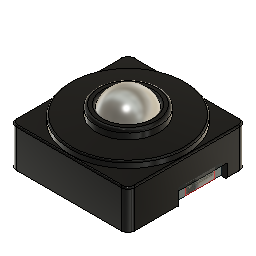
Pixart PAW3204 0A v2 (Autodesk Fusion 360 design; units mm, degrees)
Autodesk Fusion 360 part; units mm, degrees
note: some values were not read from the file. Set by a fixed rule: which sketch regions a step uses.
sketch "Skizze1" plane through (0, 0, 0) normal (0, 0, 1) x (1, 0, 0)
  line L0 (8.5, -8.5) -> (-8.5, -8.5)
  line L1 (-8.5, -8.5) -> (-8.5, 8.5)
  line L2 (-8.5, 8.5) -> (8.5, 8.5)
  line L3 (8.5, 8.5) -> (8.5, -8.5)
  line L4 (8.5, -8.5) -> (-8.5, 8.5) construction
  line L5 (-8.5, -8.5) -> (8.5, 8.5) construction
  dimension "d1" = 17
  dimension "d2" = 17
  constraint horizontal L0
  constraint perpendicular L0 L1
  constraint parallel L0 L2
  constraint parallel L1 L3
  constraint coincident L4 origin
  constraint coincident L5 origin
  measures "d1" distance of L1.end L2.end
  measures "d2" distance of L0.end L1.end
extrude "Extrusion1" add sketch "Skizze1" along normal blind 5.75 makes body 1
sketch "Skizze2" plane through (0, 0, 5.75) normal (0, 0, 1) x (-1, 0, 0)
  line L0 (-8.5, -8.5) -> (8.5, -8.5)
  line L1 (8.5, -8.5) -> (8.5, 8.5)
  line L2 (8.5, 8.5) -> (-8.5, 8.5)
  line L3 (-8.5, 8.5) -> (-8.5, -8.5)
  circle A0 centre (0, 0) radius 8.25
  dimension "d5" = 16.5
  constraint coincident A0.centre origin
  measures "d5" diameter of A0
extrude "Extrusion2" add sketch "Skizze2" along normal blind 0.9 contours A0 bodies 1
sketch "Skizze3" plane through (0, 0, 6.65) normal (0, 0, 1) x (-1, 0, 0)
  circle A0 centre (0, 0) radius 8.25
  circle A1 centre (0, 0) radius 4.5
  dimension "d8" = 9
  constraint coincident A0.centre A1.centre
  measures "d8" diameter of A1
extrude "Extrusion3" add sketch "Skizze3" along normal blind 1.25 contours A1 bodies 1
sketch "Skizze4" plane through (0, 0, 0) normal (0, 1, 0) x (1, 0, 0)
  circle A0 centre (0, -6.4) radius 3.5
  line L0 (-8.5, 0) -> (8.5, 0)
  line L1 (0, 0) -> (0, -9.9) construction
  line L2 (0, -9.9) -> (0, -2.9)
  dimension "d11" = 7
  dimension "d12" = 9.9
  constraint coincident L1.start origin
  constraint coincident A0 L1.end
  constraint coincident A0 L2.end
  constraint coincident L1 L2.end
  measures "d11" diameter of A0
  measures "d12" distance of L1.start L1.end
revolve "Drehen1" add sketch "Skizze4" angle 360 about axis through (0, 0, 0) along (0, 0, 1) separate body contours A0 L2 picked at (1.5391, -5.636) makes body 2
combine "Kombinieren1" operation cut target body 1 tool bodies 2 keep tools
fillet "Abrundung1" radius 0.3 1 edges at (-1.1435, -2.9483, 7.9) on bodies 1
fillet "Abrundung2" radius 0.4 1 edges at (4.1955, 1.6273, 7.9) on bodies 1
fillet "Abrundung3" radius 0.2 1 edges at (7.6917, 2.9833, 6.65) on bodies 1
fillet "Abrundung4" radius 1 4 edges at (-8.5, -8.5, 2.875) (8.5, -8.5, 2.875) (8.5, 8.5, 2.875) (-8.5, 8.5, 2.875) on bodies 1
fillet "Abrundung5" radius 0.2 16 edges at (-8.2071, 8.2071, 5.75) (-8.5, 0, 5.75) (-8.2071, -8.2071, 5.75) (0, -8.5, 5.75) (8.2071, -8.2071, 5.75) (8.5, 0, 5.75) (8.2071, 8.2071, 5.75) (0, 8.5, 5.75) (8.2071, 8.2071, 0) (8.5, 0, 0) (8.2071, -8.2071, 0) (0, -8.5, 0) (-8.2071, -8.2071, 0) (-8.5, 0, 0) (-8.2071, 8.2071, 0) (0, 8.5, 0) on bodies 1
sketch "Skizze5" plane through (0, 0, 0) normal (0, 0, -1) x (1, 0, 0)
  arc A0 (7.5, -8.3) -> (8.3, -7.5) centre (7.5, -7.5) ccw
  line L0 (8.3, -7.5) -> (8.3, 7.5)
  arc A1 (8.3, 7.5) -> (7.5, 8.3) centre (7.5, 7.5) ccw
  line L1 (7.5, 8.3) -> (-7.5, 8.3)
  arc A2 (-7.5, 8.3) -> (-8.3, 7.5) centre (-7.5, 7.5) ccw
  line L2 (-8.3, 7.5) -> (-8.3, -7.5)
  arc A3 (-8.3, -7.5) -> (-7.5, -8.3) centre (-7.5, -7.5) ccw
  line L3 (-7.5, -8.3) -> (7.5, -8.3)
  line L4 (8.3, 1.2) -> (6.8, 1.2)
  line L5 (6.8, 1.2) -> (6.8, -5.7)
  line L6 (6.8, -5.7) -> (8.3, -5.7)
  line L7 (8.3, -5.7) -> (8.3, 1.2)
  line L8 (6.8, 1.2) -> (9.6497, 1.2)
  line L9 (9.6497, 1.2) -> (9.6497, -5.7)
  line L10 (9.6497, -5.7) -> (6.8, -5.7)
  line L11 (6.8, -5.7) -> (6.8, 1.2)
  dimension "d24" = 9.5
  dimension "d25" = 14
  dimension "d26" = 1.5
  constraint horizontal L4
  constraint vertical L5
  constraint horizontal L6
  constraint vertical L7
  constraint collinear L0 L7
  constraint horizontal L8
  constraint vertical L9
  constraint horizontal L10
  constraint vertical L11
  constraint coincident L5.end L6.start
  measures "d24" distance of L3 L4
  measures "d25" distance of L1 L6
  measures "d26" distance of L5 L7
extrude "Extrusion4" cut sketch "Skizze5" against normal blind 2 contours L0 L4 L5 L6 L7 L8 L10 L11 | L0 L7 L8 L9 L10 bodies 1
sketch "Skizze6" plane through (0, 0, 2) normal (0, 0, -1) x (1, 0, 0)
  line L0 (8.5, -5.7) -> (8.5, 1.2)
  line L1 (8.5, 1.2) -> (6.8, 1.2)
  line L2 (6.8, 1.2) -> (6.8, -5.7)
  line L3 (6.8, -5.7) -> (8.5, -5.7)
  line L4 (7.2, 0.8) -> (7.2, -5.3)
  line L5 (7.2, -5.3) -> (8.1, -5.3)
  line L6 (8.1, -5.3) -> (8.1, 0.8)
  line L7 (8.1, 0.8) -> (7.2, 0.8)
  dimension "d30" = -0.4
extrude "Extrusion5" add sketch "Skizze6" along normal blind 1.5 separate body contours L4 L5 L6 L7 makes body 3
sketch "Skizze7" plane through (8.1, 0, 0) normal (1, 0, 0) x (0, 1, 0)
  line L0 (5.3, 2) -> (-0.8, 2)
  line L1 (-0.8, 2) -> (-0.8, 0.5)
  line L2 (-0.8, 0.5) -> (5.3, 0.5)
  line L3 (5.3, 0.5) -> (5.3, 2)
sketch "Skizze8" plane through (8.1, 0, 0) normal (1, 0, 0) x (0, 1, 0)
equation "d6 = 6.65 mm - 5.75 mm"
equation "d9 = 7.9 mm - 6.65 mm"
